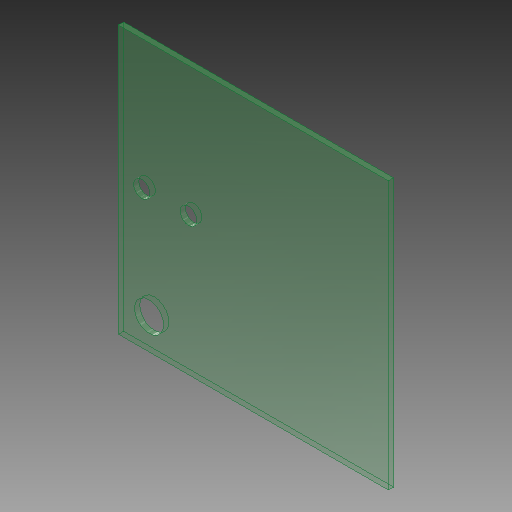
# Autodesk Inventor part: sb_side
Saved by Autodesk Inventor 2018.1 (Build 221171000, 171)
## iProperties
Created: 2017-08-17
Part Number: sb_side
Material: PVC-Piping
Document SubType Name: Modeling
Designer: Tom
Density: 1.4 g/cm^3
Appearance: Clear - Green 1
Author: Tom
Autodesk Inventor part; units mm, degrees
ref_plane "YZ Plane" through (0, 0, 0) normal (1, 0, 0) x (0, 1, 0)
ref_plane "XZ Plane" through (0, 0, 0) normal (0, 1, 0) x (-1, 0, 0)
ref_plane "XY Plane" through (0, 0, 0) normal (0, 0, 1) x (1, 0, 0)
sketch "Sketch1" plane through (0, 0, 0) normal (1, 0, 0) x (0, 1, 0)
  line L0 (-129, 130) -> (129, 130)
  line L1 (129, 130) -> (129, -130)
  line L2 (129, -130) -> (-129, -130)
  line L3 (-129, -130) -> (-129, 130)
  line L4 (-129, 130) -> (129, -130) construction
  line L5 (129, 130) -> (-129, -130) construction
  point P0 (0, 0)
  dimension "d0" = 258
  dimension "d1" = 260
  constraints: 12 end point, 2 midpoint, 2 parallel, 1 horizontal, 1 perpendicular
  measures "d0" distance of L1.end L2.end
  measures "d1" distance of L0.end L1.end
extrude "Extrusion1" add sketch "Sketch1" along normal mid plane 5
sketch "Sketch3" plane through (-2.5, 0, 0) normal (-1, 0, 0) x (0, 0, 1)
  circle A0 centre (100.5, -99.5) radius 16.7557 construction
  line L0 (130, -129) -> (130, 129) construction
  line L1 (-130, -129) -> (130, -129) construction
  circle A1 centre (100.5, -99.5) radius 14
  point P0 (0, 0)
  dimension "d12" = 29.5
  dimension "d13" = 29.5
  dimension "d14" = 28
  constraints: 2 centre point, 1 coincident
  measures "d12" distance from line of L0 A0.centre
  measures "d13" distance from line of L1 A0.centre
  measures "d14" diameter of A1
extrude "Extrusion3" cut sketch "Sketch3" against normal blind 5
sketch "Sketch4" plane through (-2.5, 0, 0) normal (-1, 0, 0) x (0, 0, 1)
  circle A0 centre (107.5, 3.5) radius 12.5 construction
  line L0 (130, -129) -> (130, 129) construction
  line L1 (-130, -129) -> (130, -129) construction
  circle A1 centre (107.5, 3.5) radius 8
  circle A2 centre (62.5, 3.5) radius 12.5 construction
  circle A3 centre (62.5, 3.5) radius 8
  point P0 (0, 0)
  dimension "d17" = 25
  dimension "d18" = 22.5
  dimension "d19" = 132.5
  dimension "d20" = 16
  dimension "d21" = 25
  dimension "d22" = 45
  dimension "d23" = 16
  dimension "d24" = 132.5
  constraints: 4 centre point, 2 coincident
  measures "d17" diameter of A0
  measures "d18" distance from line of L0 A0.centre
  measures "d19" distance from line of L1 A0.centre
  measures "d20" diameter of A1
  measures "d21" diameter of A2
  measures "d22" distance of A0.centre A2.centre
  measures "d23" diameter of A3
  measures "d24" distance from line of L1 A2.centre
extrude "Extrusion4" cut sketch "Sketch4" against normal blind 5
equation "\"d0\" = boxh"
equation "\"d1\" = boxl + 2 * pvct"
equation "\"d2\" = pvct"
equation "\"d14\" = airininner"
equation "\"d15\" = pvct"
equation "\"d17\" = diapowerouter"
equation "\"d20\" = diapower"
equation "\"d21\" = diapowerouter"
equation "\"d23\" = diapower"
equation "\"d25\" = pvct"
equation "\"solhole\" = 3"
equation "\"solholespacing\" = 16"
equation "\"ssolw\" = 63"
equation "\"bsoll\" = 126"
equation "\"bsolw\" = 91"
equation "\"bsolh\" = 126"
equation "\"tapl\" = 31"
equation "\"tl\" = 32"
equation "\"eloboww\" = 25"
equation "\"pvct\" = 5"
equation "\"boxh\" = 258"
equation "\"supporth\" = 15"
equation "\"play\" = 0.5"
equation "\"pcbh\" = 46"
equation "\"pcbw\" = 76"
equation "\"pcbl\" = 86"
equation "\"arl\" = 102"
equation "\"arw\" = 54"
equation "\"psuh\" = 85"
equation "\"screenl\" = 115"
equation "\"screenw\" = 197"
equation "\"seph\" = 105"
equation "\"diapowerouter\" = 25"
equation "\"dialoadouter\" = 25"
equation "\"distpumps\" = 75"
equation "\"diaetapeouter\" = 36"
equation "\"diaphouter\" = 48"
equation "\"distbubblewater\" = 82"
equation "\"diaload\" = 16"
equation "\"diaetape\" = 25"
equation "\"diaph\" = 32"
equation "\"diapower\" = 16"
equation "\"pumpouter\" = 25"
equation "\"airoutinner\" = 28"
equation "\"airoutouter\" = 39"
equation "\"waterouter\" = 39"
equation "\"waterinner\" = 28"
equation "\"pumpinner\" = 16"
equation "\"airininner\" = 28"
equation "\"airinouter\" = 39"
equation "\"boxl\" = 250"
body "Solid1"
